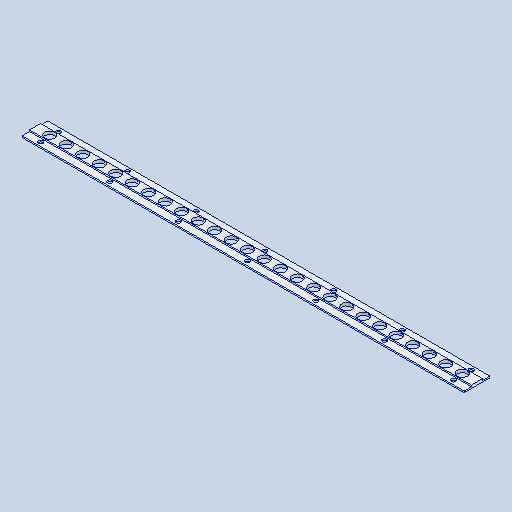
# Autodesk Inventor part: link2plate2
Saved by Autodesk Inventor 2024 (Build 280153000, 153)
## iProperties
Created: 2025-02-07
Part Number: link2plate2
Material: アルミニウム 6061
Document SubType Name: Modeling
Designer: tanoue_kota
Density: 2.7 g/cm^3
Appearance: アルミニウム - フラット
Mass: 14.5615 g
Surface Area: 108.174 cm^2
Volume: 5.39314 cm^3
Author: tanoue_kota
Autodesk Inventor part; units mm, degrees
ref_plane "YZ Plane" through (0, 0, 0) normal (1, 0, 0) x (0, 1, 0)
ref_plane "XZ Plane" through (0, 0, 0) normal (0, 1, 0) x (-1, 0, 0)
ref_plane "XY Plane" through (0, 0, 0) normal (0, 0, 1) x (1, 0, 0)
sketch "スケッチ1" plane through (0, 0, 0) normal (0, 1, 0) x (-1, 0, 0)
  line L0 (0, 0) -> (-300, 0)
  line L1 (-300, 0) -> (-300, -17.5)
  line L2 (-300, -17.5) -> (0, -17.5)
  line L3 (0, -17.5) -> (0, 0)
  dimension "d0" = 300
  dimension "d1" = 17.5
  constraints: 8 end point, 2 parallel, 1 horizontal, 1 perpendicular
  measures "d0" distance of L1.end L2.end
  measures "d1" distance of L0.end L1.end
extrude "押し出し1" add sketch "スケッチ1" along normal blind 2
sketch "スケッチ2" plane through (0, 2, 0) normal (0, 1, 0) x (1, 0, 0)
  line L0 (0, 17.5) -> (0, 0) projected
  line L1 (0, 8.75) -> (300, 8.75)
  line L2 (300, 0) -> (300, 17.5) projected
  line L3 (0, 8.75) -> (300, 8.75)
  line L4 (300, 8.75) -> (300, 12.5)
  line L5 (300, 12.5) -> (0, 12.5)
  line L6 (0, 12.5) -> (0, 8.75)
  line L7 (0, 0) -> (0, 17.5)
  line L8 (300, 17.5) -> (300, 0)
  line L9 (300, 5) -> (0, 5)
  line L10 (0, 0) -> (300, 0)
  line L11 (300, 0) -> (300, 17.5)
  line L12 (300, 17.5) -> (0, 17.5)
  line L13 (0, 17.5) -> (0, 0)
  point P0 (0, 12.5)
  point P1 (0, 5)
  dimension "d4" = 3.75
  constraints: 24 end point, 6 symmetric about line, 4 parallel, 2 horizontal, 2 midpoint, 2 perpendicular, 2 point on line
  measures "d4" distance between parallel lines of L1 L5
extrude "押し出し2" cut sketch "スケッチ2" against normal blind 1 contours L12 L2 L5 L0 | L9 L2 L10 L0
sketch "スケッチ3" plane through (0, 1, 0) normal (0, 1, 0) x (1, 0, 0)
  line L0 (300, 5) -> (300, 12.5) projected
  line L1 (300, 8.75) -> (0, 8.75)
  line L2 (0, 12.5) -> (0, 5) projected
  line L3 (0, 5) -> (300, 5) projected
  line L4 (0, 0) -> (0, 5) projected
  point P0 (10, 2.75)
  point P1 (10, 14.75)
  point P2 (56.6667, 2.75)
  point P3 (103.3333, 2.75)
  point P4 (150, 2.75)
  point P5 (196.6667, 2.75)
  point P6 (243.3333, 2.75)
  point P7 (290, 2.75)
  point P8 (56.6667, 14.75)
  point P9 (103.3333, 14.75)
  point P10 (150, 14.75)
  point P11 (196.6667, 14.75)
  point P12 (243.3333, 14.75)
  point P13 (290, 14.75)
  dimension "d42" = 10
  dimension "d43" = 6
  dimension "d46" = 46.6667
  constraints: 7 symmetric about line, 2 end point, 2 midpoint, 1 horizontal, 6 other
  measures "d42" distance from line of L4 point (10, 2.75)
  measures "d43" distance from line of L1 point (10, 2.75)
  measures "d46" distance of point (10, 2.75) point (56.667, 2.75)
hole "穴1" at (10, 1, -2.75) at (10, 1, -14.75) at (290, 1, -2.75) at (290, 1, -14.75) at (243.3333, 1, -2.75) at (243.3333, 1, -14.75) at (196.6667, 1, -14.75) at (196.6667, 1, -2.75) at (150, 1, -2.75) at (150, 1, -14.75) at (103.3333, 1, -14.75) at (103.3333, 1, -2.75) at (56.6667, 1, -14.75) at (56.6667, 1, -2.75) direction (0, -1, 0) diameter 3.1 end through all
sketch "スケッチ4" plane through (0, 2, 0) normal (0, 1, 0) x (1, 0, 0)
  line L0 (300, 0) -> (300, 17.5) projected
  line L1 (300, 8.75) -> (0, 8.75)
  line L2 (0, 12.5) -> (0, 5) projected
  point P0 (0, 0)
  point P1 (290, 8.75)
  point P2 (278.8, 8.75)
  point P3 (267.6, 8.75)
  point P4 (256.4, 8.75)
  point P5 (245.2, 8.75)
  point P6 (234, 8.75)
  point P7 (222.8, 8.75)
  point P8 (211.6, 8.75)
  point P9 (200.4, 8.75)
  point P10 (189.2, 8.75)
  point P11 (178, 8.75)
  point P12 (166.8, 8.75)
  point P13 (155.6, 8.75)
  point P14 (144.4, 8.75)
  point P15 (133.2, 8.75)
  point P16 (122, 8.75)
  point P17 (110.8, 8.75)
  point P18 (99.6, 8.75)
  point P19 (88.4, 8.75)
  point P20 (77.2, 8.75)
  point P21 (66, 8.75)
  point P22 (54.8, 8.75)
  point P23 (10, 8.75)
  point P24 (43.6, 8.75)
  point P25 (32.4, 8.75)
  point P26 (21.2, 8.75)
  dimension "d23" = 10
  dimension "d26" = 11.2
  dimension "d39" = 10
  constraints: 2 end point, 2 midpoint, 2 point on line, 1 horizontal, 24 other
  measures "d23" distance from line of L0 point (290, 8.75)
  measures "d26" distance of point (290, 8.75) point (278.8, 8.75)
  measures "d39" distance from line of L2 point (10, 8.75)
hole "穴2" at (290, 2, -8.75) at (278.8, 2, -8.75) at (267.6, 2, -8.75) at (256.4, 2, -8.75) at (245.2, 2, -8.75) at (234, 2, -8.75) at (222.8, 2, -8.75) at (211.6, 2, -8.75) at (200.4, 2, -8.75) at (189.2, 2, -8.75) at (178, 2, -8.75) at (166.8, 2, -8.75) at (155.6, 2, -8.75) at (144.4, 2, -8.75) at (133.2, 2, -8.75) at (122, 2, -8.75) at (110.8, 2, -8.75) at (99.6, 2, -8.75) at (88.4, 2, -8.75) at (77.2, 2, -8.75) at (66, 2, -8.75) at (54.8, 2, -8.75) at (10, 2, -8.75) at (43.6, 2, -8.75) at (32.4, 2, -8.75) at (21.2, 2, -8.75) direction (0, -1, 0) diameter 7 depth 8 tip angle 118
equation "\"d0\" = polygon2_len1"
equation "\"d4\" = 0.5 * polygon2_wid2"
equation "\"polygon2_len1\" = 300"
equation "\"polygon2_wid2\" = 7.5"
